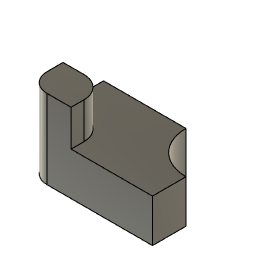
7.3 Include 3D (Autodesk Fusion 360 design; units mm, degrees)
Autodesk Fusion 360 part; units mm, degrees
sketch "Sketch1" plane through (0, 0, 0) normal (0, 0, 1) x (1, 0, 0)
  line L0 (0, 0) -> (53.9524, 0)
  line L1 (53.9524, 0) -> (53.9524, 14.5545)
  line L2 (35.7878, 32.7191) -> (0, 32.7191)
  line L3 (0, 32.7191) -> (0, 0)
  arc A0 (35.7878, 32.7191) -> (53.9524, 14.5545) centre (53.9524, 32.7191) ccw
  constraint horizontal L0
  constraint vertical L1
  constraint horizontal L2
  constraint vertical L3
  constraint coincident L0.start L3.end
extrude "Extrude1" add sketch "Sketch1" along normal blind 18.598
sketch "Sketch2" plane through (0, 0, 18.598) normal (0, 0, 1) x (-1, 0, 0)
  line L0 (0, 0) -> (-18.618, 0)
  line L1 (-18.618, 0) -> (-18.618, -15.1183)
  line L2 (-18.618, -15.1183) -> (0, -15.1183)
  line L3 (0, -15.1183) -> (0, 0)
  constraint horizontal L0
  constraint vertical L1
  constraint horizontal L2
  constraint vertical L3
  constraint coincident L0.start L3.end
extrude "Extrude2" add sketch "Sketch2" along normal blind 15.729
fillet "Fillet1" radius 9.525 1 edges at (18.618, 15.1183, 26.4625)
fillet "Fillet2" radius 8.158 1 edges at (0, 0, 17.1635)
ref_plane "WorkPlane1" through (0, 0, 45.086) normal (0, 0, 1) x (1, 0, 0)
